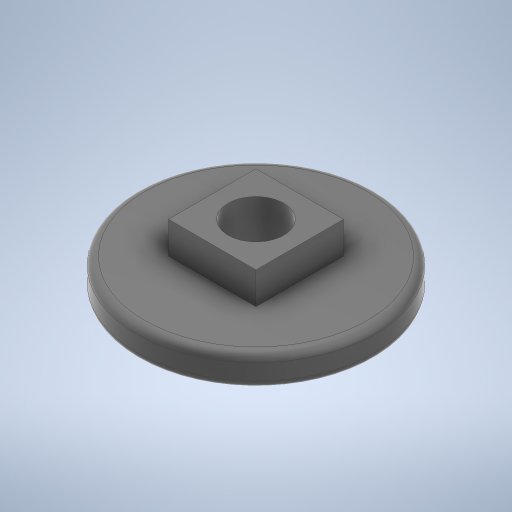
# Autodesk Inventor part: FrictionCap
Saved by Autodesk Inventor 2024 (Build 280153000, 153)
## iProperties
Created: 2026-01-10
Part Number: FrictionCap
Material: Generic
Document SubType Name: Modeling
Designer: Liam
Density: 1 g/cm^3
Appearance: Default
Author: Liam
Autodesk Inventor part; units mm, degrees
ref_plane "YZ Plane" through (0, 0, 0) normal (1, 0, 0) x (0, 1, 0)
ref_plane "XZ Plane" through (0, 0, 0) normal (0, 1, 0) x (-1, 0, 0)
ref_plane "XY Plane" through (0, 0, 0) normal (0, 0, 1) x (1, 0, 0)
sketch "Sketch1" plane through (0, 0, 0) normal (0, 1, 0) x (-1, 0, 0)
  circle A0 centre (0, 0) radius 1.75
  circle A1 centre (0, 0) radius 7.5
  line L0 (-2.75, -2.75) -> (2.75, -2.75)
  line L1 (2.75, -2.75) -> (2.75, 2.75)
  line L2 (2.75, 2.75) -> (-2.75, 2.75)
  line L3 (-2.75, 2.75) -> (-2.75, -2.75)
  line L4 (-2.75, -2.75) -> (2.75, 2.75) construction
  line L5 (2.75, -2.75) -> (-2.75, 2.75) construction
  dimension "d1" = 3.5
  dimension "d2" = 15
  dimension "d3" = 5.5
  dimension "d4" = 5.5
  constraints: 12 end point, 2 centre point, 2 coincident, 2 midpoint, 2 parallel, 1 horizontal, 1 perpendicular
  measures "d1" diameter of A0
  measures "d2" diameter of A1
  measures "d3" distance of L0.end L1.end
  measures "d4" distance of L0.start L0.end
extrude "Extrusion1" add sketch "Sketch1" along normal blind 2 contours L3 L2 L1 L0
extrude "Extrusion2" add sketch "Sketch1" against normal blind 2 contours A1 | L3 L2 L1 L0
fillet "Fillet1" radius 0.5 2 edges at (7.5, 0, 0) (7.5, -2, 0)
equation "\"d2\" = CapDiameter"
equation "\"d5\" = PIVOT_DEPTH"
equation "\"d7\" = CapHeight"
equation "\"CapDiameter\" = 15"
equation "\"CapHeight\" = 2"
equation "\"PIVOT_DEPTH\" = 2"
body "Solid1"
